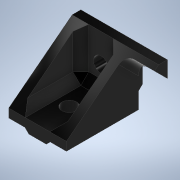
# Autodesk Inventor part: Soporte Actuador
Saved by Autodesk Inventor 2020.3 (Build 243373000, 373)
## iProperties
Created: 2021-03-04
Part Number: Soporte Actuador
Material: PET Plastic
Document SubType Name: Modeling
Designer: juanp
Density: 1.541 g/cm^3
Appearance: Polycarbonate - Clear
Author: juanp
Autodesk Inventor part; units mm, degrees
ref_plane "YZ Plane" through (0, 0, 0) normal (1, 0, 0) x (0, 1, 0)
ref_plane "XZ Plane" through (0, 0, 0) normal (0, 1, 0) x (-1, 0, 0)
ref_plane "XY Plane" through (0, 0, 0) normal (0, 0, 1) x (1, 0, 0)
sketch "Sketch1" plane through (0, 0, 0) normal (0, 1, 0) x (-1, 0, 0)
  line L0 (0, 0) -> (20, 0)
  line L1 (20, 0) -> (20, -25)
  line L2 (20, -25) -> (0, -25)
  line L3 (0, -25) -> (0, 0)
  circle A0 centre (10, -11) radius 2.6
  line L4 (20, -25) -> (0, -25)
  line L5 (0, -25) -> (0, -22)
  line L6 (0, -22) -> (20, -22)
  line L7 (20, -22) -> (20, -25)
  line L8 (0, -22) -> (20, 0) construction
  point P0 (10, -11)
  dimension "d2" = 20
  dimension "d3" = 25
  dimension "d4" = 5.2
  dimension "d7" = 3
  constraints: 18 end point, 4 parallel, 3 coincident, 2 horizontal, 2 perpendicular, 1 centre point, 1 midpoint, 1 point on line
  measures "d2" distance of L1.end L2.end
  measures "d3" distance of L0.end L1.end
  measures "d4" diameter of A0
  measures "d7" distance between parallel lines of L2 L6
extrude "Extrusion1" add sketch "Sketch1" along normal blind 3
extrude "Extrusion2" add sketch "Sketch1" along normal blind 20 contours L6 L1 L2 L3
sketch "Sketch2" plane through (0, 0, -25) normal (0, 0, -1) x (-1, 0, 0)
  line L0 (0, 0) -> (0, 20) projected
  line L1 (20, 0) -> (20, 20) projected
  line L2 (0, 20) -> (20, 0) construction
  circle A0 centre (10, 10) radius 2.65
  dimension "d10" = 5.3
  constraints: 2 end point, 1 centre point, 1 midpoint
  measures "d10" diameter of A0
extrude "Extrusion3" cut sketch "Sketch2" against normal through all
ref_plane "Work Plane1" through (-20, 20, -22) normal (0, -0.791285, -0.6114475) x (1, 0, 0)
sketch "Sketch3" plane through (-20, 20, -22) normal (0, -0.791285, -0.6114475) x (1, 0, 0)
  line L0 (0, 27.8029) -> (20, 27.8029) projected
  line L1 (0, 0) -> (20, 0) projected
  line L2 (0, 10.3946) -> (0, 0) projected
  line L3 (0, 0) -> (3, 0)
  line L4 (3, 0) -> (3, 27.8029)
  line L5 (3, 27.8029) -> (0, 27.8029)
  line L6 (0, 27.8029) -> (0, 0)
  line L7 (20, 27.8029) -> (17, 27.8029)
  line L8 (17, 27.8029) -> (17, 0)
  line L9 (17, 0) -> (20, 0)
  line L10 (20, 0) -> (20, 27.8029)
  point P0 (20, 29.6372)
  point P1 (20, 0)
  dimension "d13" = 3
  dimension "d14" = 3
  constraints: 16 end point, 4 parallel, 2 horizontal, 2 perpendicular, 2 point on line
  measures "d13" distance between parallel lines of L2 L4
  measures "d14" distance between parallel lines of L10 L8
extrude "Extrusion4" add sketch "Sketch3" along normal up to next contours L0 L4 L1 L2 L6 | L0 L10 L1 L8
chamfer "Chamfer1" distance 2.75 angle 45 5 edges at (-10, 3, -22) (-3, 11.5, -22) (-3, 3, -11) (-17, 3, -11) (-17, 11.5, -22)
sketch "Sketch4" plane through (0, 0, 0) normal (0, -1, 0) x (1, 0, 0)
  line L0 (0, -25) -> (-20, -25) projected
  line L1 (-20, 0) -> (0, 0) projected
  line L2 (-14.375, -25) -> (-5.625, -25)
  line L3 (-5.625, -25) -> (-5.625, 0)
  line L4 (-5.625, 0) -> (-14.375, 0)
  line L5 (-14.375, 0) -> (-14.375, -25)
  circle A0 centre (-10, -11) radius 2.6 projected
  line L6 (-10, -25) -> (-10, 0) construction
  point P0 (-14.375, 0)
  dimension "d32" = 8.75
  constraints: 10 end point, 3 point on line, 2 midpoint, 2 parallel, 1 horizontal, 1 perpendicular
  measures "d32" distance between parallel lines of L5 L3
extrude "Extrusion5" add sketch "Sketch4" along normal blind 1.35
sketch "Sketch5" plane through (0, 20, -25) normal (0, 0, -1) x (-1, 0, 0)
  line L0 (0, 0) -> (0, -17) projected
  line L1 (20, -17) -> (20, 0) projected
  line L2 (0, -5.625) -> (20, -5.625)
  line L3 (20, -5.625) -> (20, -14.375)
  line L4 (20, -14.375) -> (0, -14.375)
  line L5 (0, -14.375) -> (0, -5.625)
  line L6 (0, -14.375) -> (20, -5.625) construction
  circle A0 centre (10, -10) radius 2.65 projected
  point P0 (0, -20)
  point P1 (0, -14.375)
  dimension "d26" = 8.75
  constraints: 10 end point, 2 parallel, 2 point on line, 1 coincident, 1 horizontal, 1 midpoint, 1 perpendicular
  measures "d26" distance between parallel lines of L2 L4
extrude "Extrusion6" add sketch "Sketch5" along normal blind 1.35
chamfer "Chamfer2" distance 1.35 angle 45 4 edges at (-10, 5.625, -26.35) (-10, 14.375, -26.35) (-14.375, -1.35, -12.5) (-5.625, -1.35, -12.5)
sketch "Sketch8" plane through (0, 0, 0) normal (1, 0, 0) x (0, 0, -1)
  line L0 (25, 14.375) -> (26.35, 13.025) projected
  line L1 (25, 14.375) -> (25, 20) projected
  line L2 (22, 20) -> (25, 20) projected
  line L3 (22, 20) -> (0, 3) projected
  line L4 (0, 0) -> (0, 3) projected
  line L5 (0, 0) -> (25, 0) projected
  line L6 (25, 0) -> (25, 5.625) projected
  line L7 (26.35, 6.975) -> (25, 5.625) projected
  line L8 (26.35, 13.025) -> (26.35, 6.975) projected
  line L9 (22, 20) -> (19.25, 17.875) projected
  line L10 (25, 14.375) -> (20.5192, 18.8558)
  line L11 (25, 14.375) -> (26.35, 13.025) projected
  constraints: 2 end point, 1 collinear, 1 point on line
extrude "Extrusion9" add sketch "Sketch8" along normal blind 10 contours L10 L3 L2 L1
fillet "Fillet1" radius 3 1 edges at (0, 16.6154, -22.7596)
body "Solid1"
